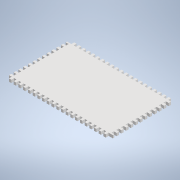
# Autodesk Inventor part: top
Saved by Autodesk Inventor 2022 (Build 260153000, 153)
## iProperties
Created: 2023-05-26
Part Number: top
Material: Типовые
Document SubType Name: Modeling
Designer: korsh624
Density: 1 g/cm^3
Appearance: По умолчанию
Author: korsh624
Autodesk Inventor part; units mm, degrees
ref_plane "YZ Plane" through (0, 0, 0) normal (1, 0, 0) x (0, 1, 0)
ref_plane "XZ Plane" through (0, 0, 0) normal (0, 1, 0) x (-1, 0, 0)
ref_plane "XY Plane" through (0, 0, 0) normal (0, 0, 1) x (1, 0, 0)
sketch "Эскиз1" plane through (0, 0, 0) normal (0, 1, 0) x (-1, 0, 0)
  line L0 (0, 0) -> (208, 0)
  line L1 (208, 0) -> (208, 123)
  line L2 (208, 123) -> (0, 123)
  line L3 (0, 123) -> (0, 0)
  line L4 (208, 125) -> (208, 130)
  line L5 (208, 123) -> (214, 123)
  line L6 (214, 123) -> (214, 118)
  line L7 (214, 118) -> (208, 118)
  line L8 (208, 118) -> (208, 123)
  line L9 (208, 113) -> (214, 113)
  line L10 (214, 113) -> (214, 108)
  line L11 (214, 108) -> (208, 108)
  line L12 (208, 108) -> (208, 113)
  line L13 (208, 103) -> (214, 103)
  line L14 (214, 103) -> (214, 98)
  line L15 (214, 98) -> (208, 98)
  line L16 (208, 98) -> (208, 103)
  line L17 (208, 93) -> (214, 93)
  line L18 (214, 93) -> (214, 88)
  line L19 (214, 88) -> (208, 88)
  line L20 (208, 88) -> (208, 93)
  line L21 (208, 83) -> (214, 83)
  line L22 (214, 83) -> (214, 78)
  line L23 (214, 78) -> (208, 78)
  line L24 (208, 78) -> (208, 83)
  line L25 (208, 73) -> (214, 73)
  line L26 (214, 73) -> (214, 68)
  line L27 (214, 68) -> (208, 68)
  line L28 (208, 68) -> (208, 73)
  line L29 (208, 63) -> (214, 63)
  line L30 (214, 63) -> (214, 58)
  line L31 (214, 58) -> (208, 58)
  line L32 (208, 58) -> (208, 63)
  line L33 (208, 53) -> (214, 53)
  line L34 (214, 53) -> (214, 48)
  line L35 (214, 48) -> (208, 48)
  line L36 (208, 48) -> (208, 53)
  line L37 (208, 43) -> (214, 43)
  line L38 (214, 43) -> (214, 38)
  line L39 (214, 38) -> (208, 38)
  line L40 (208, 38) -> (208, 43)
  line L41 (208, 33) -> (214, 33)
  line L42 (214, 33) -> (214, 28)
  line L43 (214, 28) -> (208, 28)
  line L44 (208, 28) -> (208, 33)
  line L45 (208, 23) -> (214, 23)
  line L46 (214, 23) -> (214, 18)
  line L47 (214, 18) -> (208, 18)
  line L48 (208, 18) -> (208, 23)
  line L49 (208, 13) -> (214, 13)
  line L50 (214, 13) -> (214, 8)
  line L51 (214, 8) -> (208, 8)
  line L52 (208, 8) -> (208, 13)
  line L53 (208, 3) -> (214, 3)
  line L54 (214, 3) -> (214, -2)
  line L55 (214, -2) -> (208, -2)
  line L56 (208, -2) -> (208, 3)
  line L57 (208, 3) -> (214, 3)
  line L58 (214, 3) -> (214, 0)
  line L59 (214, 0) -> (208, 0)
  line L60 (208, 0) -> (208, 3)
  line L61 (0, 0) -> (-6, 0)
  line L62 (-6, 0) -> (-6, 5)
  line L63 (-6, 5) -> (0, 5)
  line L64 (0, 5) -> (0, 0)
  line L65 (0, 15) -> (0, 10)
  line L66 (0, 10) -> (-6, 10)
  line L67 (-6, 10) -> (-6, 15)
  line L68 (-6, 15) -> (0, 15)
  line L69 (0, 25) -> (0, 20)
  line L70 (0, 20) -> (-6, 20)
  line L71 (-6, 20) -> (-6, 25)
  line L72 (-6, 25) -> (0, 25)
  line L73 (0, 35) -> (0, 30)
  line L74 (0, 30) -> (-6, 30)
  line L75 (-6, 30) -> (-6, 35)
  line L76 (-6, 35) -> (0, 35)
  line L77 (0, 45) -> (0, 40)
  line L78 (0, 40) -> (-6, 40)
  line L79 (-6, 40) -> (-6, 45)
  line L80 (-6, 45) -> (0, 45)
  line L81 (0, 55) -> (0, 50)
  line L82 (0, 50) -> (-6, 50)
  line L83 (-6, 50) -> (-6, 55)
  line L84 (-6, 55) -> (0, 55)
  line L85 (0, 65) -> (0, 60)
  line L86 (0, 60) -> (-6, 60)
  line L87 (-6, 60) -> (-6, 65)
  line L88 (-6, 65) -> (0, 65)
  line L89 (0, 75) -> (0, 70)
  line L90 (0, 70) -> (-6, 70)
  line L91 (-6, 70) -> (-6, 75)
  line L92 (-6, 75) -> (0, 75)
  line L93 (0, 85) -> (0, 80)
  line L94 (0, 80) -> (-6, 80)
  line L95 (-6, 80) -> (-6, 85)
  line L96 (-6, 85) -> (0, 85)
  line L97 (0, 95) -> (0, 90)
  line L98 (0, 90) -> (-6, 90)
  line L99 (-6, 90) -> (-6, 95)
  line L100 (-6, 95) -> (0, 95)
  line L101 (0, 105) -> (0, 100)
  line L102 (0, 100) -> (-6, 100)
  line L103 (-6, 100) -> (-6, 105)
  line L104 (-6, 105) -> (0, 105)
  line L105 (0, 115) -> (0, 110)
  line L106 (0, 110) -> (-6, 110)
  line L107 (-6, 110) -> (-6, 115)
  line L108 (-6, 115) -> (0, 115)
  line L109 (0, 125) -> (0, 120)
  line L110 (0, 120) -> (-6, 120)
  line L111 (-6, 120) -> (-6, 125)
  line L112 (-6, 125) -> (0, 125)
  line L113 (0, 120) -> (-6, 120)
  line L114 (-6, 120) -> (-6, 123)
  line L115 (-6, 123) -> (0, 123)
  line L116 (0, 123) -> (0, 120)
  line L117 (208, 123) -> (203, 123)
  line L118 (203, 123) -> (203, 129)
  line L119 (203, 129) -> (208, 129)
  line L120 (208, 129) -> (208, 123)
  line L121 (198, 125) -> (198, 130)
  line L122 (198, 123) -> (193, 123)
  line L123 (198, 129) -> (198, 123)
  line L124 (193, 129) -> (198, 129)
  line L125 (193, 123) -> (193, 129)
  line L126 (188, 125) -> (188, 130)
  line L127 (188, 123) -> (183, 123)
  line L128 (188, 129) -> (188, 123)
  line L129 (183, 129) -> (188, 129)
  line L130 (183, 123) -> (183, 129)
  line L131 (178, 125) -> (178, 130)
  line L132 (178, 123) -> (173, 123)
  line L133 (178, 129) -> (178, 123)
  line L134 (173, 129) -> (178, 129)
  line L135 (173, 123) -> (173, 129)
  line L136 (168, 125) -> (168, 130)
  line L137 (168, 123) -> (163, 123)
  line L138 (168, 129) -> (168, 123)
  line L139 (163, 129) -> (168, 129)
  line L140 (163, 123) -> (163, 129)
  line L141 (158, 125) -> (158, 130)
  line L142 (158, 123) -> (153, 123)
  line L143 (158, 129) -> (158, 123)
  line L144 (153, 129) -> (158, 129)
  line L145 (153, 123) -> (153, 129)
  line L146 (148, 125) -> (148, 130)
  line L147 (148, 123) -> (143, 123)
  line L148 (148, 129) -> (148, 123)
  line L149 (143, 129) -> (148, 129)
  line L150 (143, 123) -> (143, 129)
  line L151 (138, 125) -> (138, 130)
  line L152 (138, 123) -> (133, 123)
  line L153 (138, 129) -> (138, 123)
  line L154 (133, 129) -> (138, 129)
  line L155 (133, 123) -> (133, 129)
  line L156 (128, 125) -> (128, 130)
  line L157 (128, 123) -> (123, 123)
  line L158 (128, 129) -> (128, 123)
  line L159 (123, 129) -> (128, 129)
  line L160 (123, 123) -> (123, 129)
  line L161 (118, 125) -> (118, 130)
  line L162 (118, 123) -> (113, 123)
  line L163 (118, 129) -> (118, 123)
  line L164 (113, 129) -> (118, 129)
  line L165 (113, 123) -> (113, 129)
  line L166 (108, 125) -> (108, 130)
  line L167 (108, 123) -> (103, 123)
  line L168 (108, 129) -> (108, 123)
  line L169 (103, 129) -> (108, 129)
  line L170 (103, 123) -> (103, 129)
  line L171 (98, 125) -> (98, 130)
  line L172 (98, 123) -> (93, 123)
  line L173 (98, 129) -> (98, 123)
  line L174 (93, 129) -> (98, 129)
  line L175 (93, 123) -> (93, 129)
  line L176 (88, 125) -> (88, 130)
  line L177 (88, 123) -> (83, 123)
  line L178 (88, 129) -> (88, 123)
  line L179 (83, 129) -> (88, 129)
  line L180 (83, 123) -> (83, 129)
  line L181 (78, 125) -> (78, 130)
  line L182 (78, 123) -> (73, 123)
  line L183 (78, 129) -> (78, 123)
  line L184 (73, 129) -> (78, 129)
  line L185 (73, 123) -> (73, 129)
  line L186 (68, 125) -> (68, 130)
  line L187 (68, 123) -> (63, 123)
  line L188 (68, 129) -> (68, 123)
  line L189 (63, 129) -> (68, 129)
  line L190 (63, 123) -> (63, 129)
  line L191 (58, 125) -> (58, 130)
  line L192 (58, 123) -> (53, 123)
  line L193 (58, 129) -> (58, 123)
  line L194 (53, 129) -> (58, 129)
  line L195 (53, 123) -> (53, 129)
  line L196 (48, 125) -> (48, 130)
  line L197 (48, 123) -> (43, 123)
  line L198 (48, 129) -> (48, 123)
  line L199 (43, 129) -> (48, 129)
  line L200 (43, 123) -> (43, 129)
  line L201 (38, 125) -> (38, 130)
  line L202 (38, 123) -> (33, 123)
  line L203 (38, 129) -> (38, 123)
  line L204 (33, 129) -> (38, 129)
  line L205 (33, 123) -> (33, 129)
  line L206 (28, 125) -> (28, 130)
  line L207 (28, 123) -> (23, 123)
  line L208 (28, 129) -> (28, 123)
  line L209 (23, 129) -> (28, 129)
  line L210 (23, 123) -> (23, 129)
  line L211 (18, 125) -> (18, 130)
  line L212 (18, 123) -> (13, 123)
  line L213 (18, 129) -> (18, 123)
  line L214 (13, 129) -> (18, 129)
  line L215 (13, 123) -> (13, 129)
  line L216 (8, 125) -> (8, 130)
  line L217 (8, 123) -> (3, 123)
  line L218 (8, 129) -> (8, 123)
  line L219 (3, 129) -> (8, 129)
  line L220 (3, 123) -> (3, 129)
  line L221 (0, 0) -> (5, 0)
  line L222 (5, 0) -> (5, -6)
  line L223 (5, -6) -> (0, -6)
  line L224 (0, -6) -> (0, 0)
  line L225 (10, 0) -> (15, 0)
  line L226 (10, -6) -> (10, 0)
  line L227 (15, -6) -> (10, -6)
  line L228 (15, 0) -> (15, -6)
  line L229 (20, 0) -> (25, 0)
  line L230 (20, -6) -> (20, 0)
  line L231 (25, -6) -> (20, -6)
  line L232 (25, 0) -> (25, -6)
  line L233 (30, 0) -> (35, 0)
  line L234 (30, -6) -> (30, 0)
  line L235 (35, -6) -> (30, -6)
  line L236 (35, 0) -> (35, -6)
  line L237 (40, 0) -> (45, 0)
  line L238 (40, -6) -> (40, 0)
  line L239 (45, -6) -> (40, -6)
  line L240 (45, 0) -> (45, -6)
  line L241 (50, 0) -> (55, 0)
  line L242 (50, -6) -> (50, 0)
  line L243 (55, -6) -> (50, -6)
  line L244 (55, 0) -> (55, -6)
  line L245 (60, 0) -> (65, 0)
  line L246 (60, -6) -> (60, 0)
  line L247 (65, -6) -> (60, -6)
  line L248 (65, 0) -> (65, -6)
  line L249 (70, 0) -> (75, 0)
  line L250 (70, -6) -> (70, 0)
  line L251 (75, -6) -> (70, -6)
  line L252 (75, 0) -> (75, -6)
  line L253 (80, 0) -> (85, 0)
  line L254 (80, -6) -> (80, 0)
  line L255 (85, -6) -> (80, -6)
  line L256 (85, 0) -> (85, -6)
  line L257 (90, 0) -> (95, 0)
  line L258 (90, -6) -> (90, 0)
  line L259 (95, -6) -> (90, -6)
  line L260 (95, 0) -> (95, -6)
  line L261 (100, 0) -> (105, 0)
  line L262 (100, -6) -> (100, 0)
  line L263 (105, -6) -> (100, -6)
  line L264 (105, 0) -> (105, -6)
  line L265 (110, 0) -> (115, 0)
  line L266 (110, -6) -> (110, 0)
  line L267 (115, -6) -> (110, -6)
  line L268 (115, 0) -> (115, -6)
  line L269 (120, 0) -> (125, 0)
  line L270 (120, -6) -> (120, 0)
  line L271 (125, -6) -> (120, -6)
  line L272 (125, 0) -> (125, -6)
  line L273 (130, 0) -> (135, 0)
  line L274 (130, -6) -> (130, 0)
  line L275 (135, -6) -> (130, -6)
  line L276 (135, 0) -> (135, -6)
  line L277 (140, 0) -> (145, 0)
  line L278 (140, -6) -> (140, 0)
  line L279 (145, -6) -> (140, -6)
  line L280 (145, 0) -> (145, -6)
  line L281 (150, 0) -> (155, 0)
  line L282 (150, -6) -> (150, 0)
  line L283 (155, -6) -> (150, -6)
  line L284 (155, 0) -> (155, -6)
  line L285 (160, 0) -> (165, 0)
  line L286 (160, -6) -> (160, 0)
  line L287 (165, -6) -> (160, -6)
  line L288 (165, 0) -> (165, -6)
  line L289 (170, 0) -> (175, 0)
  line L290 (170, -6) -> (170, 0)
  line L291 (175, -6) -> (170, -6)
  line L292 (175, 0) -> (175, -6)
  line L293 (180, 0) -> (185, 0)
  line L294 (180, -6) -> (180, 0)
  line L295 (185, -6) -> (180, -6)
  line L296 (185, 0) -> (185, -6)
  line L297 (190, 0) -> (195, 0)
  line L298 (190, -6) -> (190, 0)
  line L299 (195, -6) -> (190, -6)
  line L300 (195, 0) -> (195, -6)
  line L301 (200, 0) -> (205, 0)
  line L302 (200, -6) -> (200, 0)
  line L303 (205, -6) -> (200, -6)
  line L304 (205, 0) -> (205, -6)
  point P0 (208, 115)
  point P1 (208, 105)
  point P2 (208, 95)
  point P3 (208, 85)
  point P4 (208, 75)
  point P5 (208, 65)
  point P6 (208, 55)
  point P7 (208, 45)
  point P8 (208, 35)
  point P9 (208, 25)
  point P10 (208, 15)
  point P11 (208, 5)
  dimension "d0" = 123
  dimension "d1" = 208
  dimension "d5" = 6
  dimension "d6" = 5
  dimension "d9" = 10
  dimension "d14" = 6
  dimension "d15" = 5
  dimension "d18" = 10
  dimension "d23" = 5
  dimension "d24" = 6
  dimension "d27" = 10
  dimension "d32" = 5
  dimension "d33" = 6
  dimension "d36" = 10
  constraints: 602 end point, 200 horizontal alignment, 160 parallel, 128 collinear, 108 vertical alignment, 6 horizontal, 6 perpendicular, 2 point on line, 13 other
  measures "d0" distance of point (208, 0) L5.start
  measures "d1" distance of L5.start point (0, 123)
  measures "d5" distance of L6.end L7.end
  measures "d6" distance of L5.end L6.end
  measures "d9" distance of L5.start L9.start
  measures "d14" distance of L62.end L63.end
  measures "d15" distance of L61.end L62.end
  measures "d18" distance of L63.end L65.start
  measures "d23" distance of L118.end L119.end
  measures "d24" distance of L117.end L118.end
  measures "d27" distance of L5.start L122.start
  measures "d32" distance of L222.end L223.end
  measures "d33" distance of L221.end L222.end
  measures "d36" distance of L221.end L225.end
extrude "Выдавливание1" add sketch "Эскиз1" along normal blind 6 contours L3 L2 L1 L0 | L61 L62 L63 L3 | L0 L222 L223 L224 | L0 L228 L227 L226 | L66 L67 L68 L3 | L0 L232 L231 L230 | L70 L71 L72 L3 | L0 L236 L235 L234 | L74 L75 L76 L3 | L0 L240 L239 L238 | L78 L79 L80 L3 | L0 L244 L243 L242 | L82 L83 L84 L3 | L0 L248 L247 L246 | L86 L87 L88 L3 | L0 L252 L251 L250 | L90 L91 L92 L3 | L0 L256 L255 L254 | L94 L95 L96 L3 | L0 L260 L259 L258 | L98 L99 L100 L3 | L0 L264 L263 L262 | L102 L103 L104 L3 | L0 L268 L267 L266 | L106 L107 L108 L3 | L0 L272 L271 L270 | L110 L111 L115 L3 | L0 L276 L275 L274 | L220 L219 L216 L218 L2 | L0 L280 L279 L278 | L215 L214 L211 L213 L2 | L0 L284 L283 L282 | L210 L209 L206 L208 L2 | L0 L288 L287 L286 | L205 L204 L201 L203 L2 | L0 L292 L291 L290 | L200 L199 L196 L198 L2 | L0 L296 L295 L294 | L195 L194 L191 L193 L2 | L0 L300 L299 L298 | L190 L189 L186 L188 L2 | L0 L304 L303 L302 | L185 L184 L181 L183 L2 | L1 L53 L54 L59 | L180 L179 L176 L178 L2 | L1 L49 L50 L51 | L175 L174 L171 L173 L2 | L1 L45 L46 L47 | L170 L169 L166 L168 L2 | L1 L41 L42 L43 | L165 L164 L161 L163 L2 | L1 L37 L38 L39 | L160 L159 L156 L158 L2 | L1 L33 L34 L35 | L155 L154 L151 L153 L2 | L1 L29 L30 L31 | L150 L149 L146 L148 L2 | L1 L25 L26 L27 | L145 L144 L141 L143 L2 | L1 L21 L22 L23 | L140 L139 L136 L138 L2 | L1 L17 L18 L19 | L135 L134 L131 L133 L2 | L1 L13 L14 L15 | L130 L129 L126 L128 L2 | L1 L9 L10 L11 | L125 L124 L121 L123 L2 | L1 L5 L6 L7 | L118 L119 L4 L120 L2
